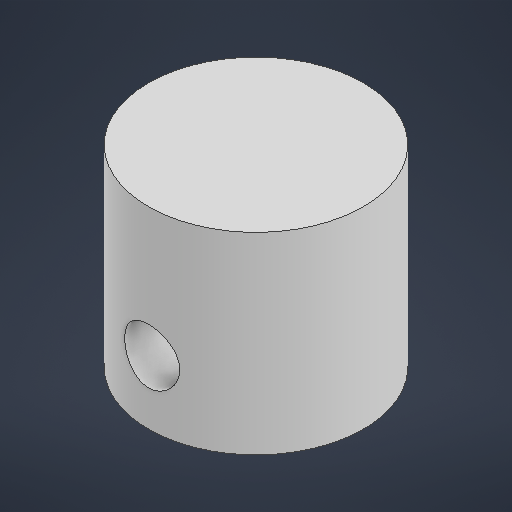
# Autodesk Inventor part: Lego_Frame_Holder
Saved by Autodesk Inventor 2025 (Build 290162010, 162A)
## iProperties
Created: 2024-06-07
Part Number: Lego_Frame_Holder
Material: Generic
Document SubType Name: Modeling
Designer: DELL
Density: 1 g/cm^3
Appearance: Default
Author: DELL
Autodesk Inventor part; units mm, degrees
ref_plane "YZ Plane" through (0, 0, 0) normal (1, 0, 0) x (0, 1, 0)
ref_plane "XZ Plane" through (0, 0, 0) normal (0, 1, 0) x (-1, 0, 0)
sketch "Sketch1" plane through (0, 0, 0) normal (0, 1, 0) x (-1, 0, 0)
  circle A0 centre (0, 0) radius 3.9
  dimension "d0" = 7.8
  constraints: 1 centre point, 1 coincident
  measures "d0" diameter of A0
extrude "Extrusion1" add sketch "Sketch1" along normal blind 7
sketch "Sketch5" plane through (0, 0, 0) normal (0, -1, 0) x (1, 0, 0)
  circle A0 centre (0, 0) radius 2.4
  dimension "d22" = 4.8
  constraints: 1 centre point, 1 coincident
  measures "d22" diameter of A0
extrude "Extrusion3" cut sketch "Sketch5" against normal blind 5
ref_plane "Work Plane1" through (0, 0, 3.9) normal (0, 0, 1) x (1, 0, 0)
sketch "Sketch2" plane through (0, 0, 3.9) normal (0, 0, 1) x (1, 0, 0)
  line L0 (0, 0) -> (0, 2.3) construction
  line L1 (3.9, 0) -> (-3.9, 0) construction
  dimension "d21" = 2.3
  constraints: 2 end point, 1 perpendicular
  measures "d21" distance of L0.start L0.end
hole "Hole1" at (0, 2.3, 3.9) direction (0, 0, -1) diameter 2 end through all
body "Solid1"
